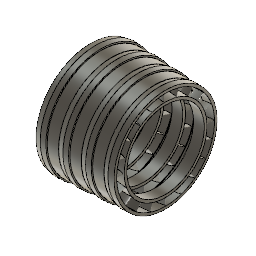
Untitled v3 (Autodesk Fusion 360 design; units mm, degrees)
Autodesk Fusion 360 part; units mm, degrees
note: some values were not read from the file. Chosen so that the rebuilt part matches the saved one: which bodies a step acts on.
sketch "Sketch1" plane through (0, 0, 0) normal (0, 1, 0) x (1, 0, 0)
  line L0 (0, -72.01) -> (20, -72.01)
  line L1 (40, -72.01) -> (60, -72.01)
  line L2 (80, -72.01) -> (100, -72.01)
  line L3 (120, -72.01) -> (140, -72.01)
  line L4 (120, -77.01) -> (140, -77.01)
  line L5 (80, -77.01) -> (100, -77.01)
  line L6 (40, -77.01) -> (60, -77.01)
  line L7 (0, -77.01) -> (20, -77.01)
  line L8 (0, -72.01) -> (234.5809, -72.01) construction
  line L9 (0, -72.01) -> (0, -77.01)
  line L10 (20, -72.01) -> (20, -77.01)
  line L11 (40, -72.01) -> (40, -77.01)
  line L12 (60, -72.01) -> (60, -77.01)
  line L13 (80, -72.01) -> (80, -77.01)
  line L14 (100, -72.01) -> (100, -77.01)
  line L15 (120, -72.01) -> (120, -77.01)
  line L16 (140, -72.01) -> (140, -77.01)
  line L17 (0, -98.8982) -> (0, -101.4021)
  line L18 (40, -96.6619) -> (40, -98.1642)
  line L19 (80, -94.4255) -> (80, -95.9279)
  line L20 (120, -92.1892) -> (120, -93.6915)
  line L21 (140, -91.071) -> (140, -121.2503)
  line L22 (140, -96.0788) -> (129.3625, -96.6736)
  line L23 (140.0185, -91.07) -> (120, -92.1892)
  line L24 (100, -98.3152) -> (90, -98.8743)
  line L25 (100, -93.3074) -> (80, -94.4255)
  line L26 (60, -100.5515) -> (50, -101.1106)
  line L27 (20, -102.7879) -> (10, -103.347)
  line L28 (60, -95.5437) -> (39.9, -96.6675)
  line L29 (20, -97.7801) -> (0, -98.8982)
  line L30 (0, 0) -> (0, -77.01) construction
  line L31 (0, -98.8982) -> (0, -101.4021) construction
  line L32 (10, -103.347) -> (0, -101.4021)
  line L33 (129.3625, -96.6736) -> (129.374, -96.6736)
  line L34 (129.374, -96.6736) -> (120, -94.6931)
  line L35 (90, -98.8743) -> (80, -96.9295)
  line L36 (50, -101.1106) -> (40, -99.1658)
  line L37 (20, -100.284) -> (40, -99.1658)
  line L38 (20, -99.2824) -> (40, -98.1642)
  line L39 (60, -98.0476) -> (80, -96.9295)
  line L40 (100, -95.8113) -> (120, -94.6931)
  line L41 (60, -97.0461) -> (80, -95.9279)
  line L42 (100, -94.8097) -> (119.9442, -93.6947)
  line L43 (100, -93.3074) -> (100, -94.8097)
  line L44 (100, -95.8113) -> (100, -115.1614)
  line L45 (119.9442, -93.6947) -> (120, -93.6915)
  line L46 (60, -95.5437) -> (60, -97.0461)
  line L47 (60, -98.0476) -> (60, -117.9989)
  line L48 (20, -97.7801) -> (20, -99.2824)
  line L49 (20, -100.284) -> (20, -102.7879)
  point P0 (160, -72.01)
  dimension "d2" = 20
  dimension "d3" = 20
  dimension "d4" = 20
  dimension "d5" = 20
  dimension "d6" = 20
  dimension "d7" = 20
  dimension "d8" = 20
  dimension "d9" = 5
  dimension "d10" = 5
  dimension "d11" = 5
  dimension "d12" = 5
  dimension "d13" = 234.5809
  dimension "d14" = 72.01
  dimension "d15" = 19.06
  dimension "d16" = 20
  dimension "d17" = 3.2
  constraint coincident L30.start origin
  constraint vertical L30
  constraint coincident L0.start L30
  constraint perpendicular L0 L30
  constraint perpendicular L8 L30
  constraint coincident L17.start L30
  constraint coincident L8 P0
  constraint coincident L29.start L23
  constraint coincident L27.start L22
  constraint parallel L10 L48
  constraint coincident L28.end L23
  constraint perpendicular L6 L18
  constraint perpendicular L6 L46
  constraint perpendicular L5 L19
  constraint perpendicular L5 L43
  constraint perpendicular L4 L20
  constraint perpendicular L4 L21
  constraint coincident L21 L22.start
  constraint coincident L24.start L43
  constraint collinear L22 L24
  constraint collinear L23 L25
  constraint coincident L26.start L46
  constraint collinear L24 L26
  constraint collinear L25 L28
  constraint collinear L26 L27
  constraint collinear L28 L29
  constraint collinear L30 L31
  constraint coincident L28 L18.start
  constraint coincident L23 L21.start
  constraint perpendicular L20 L33
  constraint coincident L35.end L39.end
  constraint coincident L36.end L37.end
  constraint parallel L35 L36
  constraint coincident L37.start L48
  constraint coincident L39.start L46
  constraint collinear L37 L39
  constraint collinear L38 L41
  constraint coincident L40.start L43
  constraint collinear L39 L40
  constraint collinear L41 L42
  constraint collinear L43 L44
  constraint parallel L42 L45
  constraint collinear L46 L47
  constraint collinear L48 L49
  measures "d2" distance of L0.start L0.end
  measures "d3" distance of L1.start L1.end
  measures "d4" distance of L2.start L2.end
  measures "d5" distance of L3.start L3.end
  measures "d6" distance of L0.end L1.start
  measures "d7" distance of L1.end L2.start
  measures "d8" distance of L2.end L3.start
  measures "d13" distance of L0.start L8.end
  measures "d14" distance of L30.start L8
  measures "d15" distance of L3.end L23.start
  measures "d16" distance of L3.end P0
  measures "d17" angle of L0 L23
revolve "Revolve1" add sketch "Sketch1" angle 360 about axis through (1.75, 0, 0) along (1, 0, 0) makes body 1 at (86.6667, 3.8386, 76.9143) makes body 2 at (46.6667, 3.8386, 76.9143) makes body 3 at (126.6667, 3.8386, 76.9143) makes body 4 at (6.6667, 3.8386, 76.9143) makes body 5 at (26.6667, 4.9802, 99.7871)
sketch "Sketch2" plane through (0, 0, 0) normal (0, 0, 1) x (1, 0, 0)
  ellipse E0 centre (10, 0) end of major axis (18.8633, -1.5628) minor radius 1
  line L0 (1.1367, 1.5628) -> (18.8633, -1.5628) construction
  line L1 (9.8264, -0.9848) -> (10.1736, 0.9848) construction
  line L2 (0, 0) -> (202.6792, 0) construction
  ellipse E1 centre (50, 0) end of major axis (58.8633, -1.5628) minor radius 1
  line L3 (41.1367, 1.5628) -> (58.8633, -1.5628) construction
  line L4 (49.8264, -0.9848) -> (50.1736, 0.9848) construction
  ellipse E2 centre (90, 0) end of major axis (98.8633, -1.5628) minor radius 1
  line L5 (81.1367, 1.5628) -> (98.8633, -1.5628) construction
  line L6 (89.8264, -0.9848) -> (90.1736, 0.9848) construction
  ellipse E3 centre (129.3716, 0) end of major axis (138.2348, -1.5628) minor radius 1
  line L7 (120.5083, 1.5628) -> (138.2348, -1.5628) construction
  line L8 (129.1979, -0.9848) -> (129.5452, 0.9848) construction
  point P0 (10, 0)
  point P1 (50, 0)
  point P2 (90, 0)
  point P3 (129.3716, 0)
  dimension "d27" = 18
  dimension "d28" = 2
  dimension "d29" = 10
  dimension "d30" = 18
  dimension "d31" = 2
  dimension "d32" = 10
  dimension "d33" = 18
  dimension "d34" = 2
  dimension "d35" = 10
  dimension "d36" = 18
  dimension "d37" = 2
  dimension "d38" = 10
  constraint coincident E0 L0.start
  constraint coincident E0 L0.end
  constraint coincident E0 L1.start
  constraint coincident E0 L1.end
  constraint coincident P0 E0.centre
  constraint coincident L2.start origin
  constraint horizontal L2
  constraint coincident E1 L3.start
  constraint coincident E1 L3.end
  constraint coincident E1 L4.start
  constraint coincident E1 L4.end
  constraint coincident P1 E1.centre
  constraint coincident E2 L5.start
  constraint coincident E2 L5.end
  constraint coincident E2 L6.start
  constraint coincident E2 L6.end
  constraint coincident P2 E2.centre
  constraint coincident E3 L7.start
  constraint coincident E3 L7.end
  constraint coincident E3 L8.start
  constraint coincident E3 L8.end
  constraint coincident P3 E3.centre
  measures "d27" distance of E0
  measures "d29" angle of L0 L2
  measures "d30" distance of E1
  measures "d32" angle of L2 L3
  measures "d33" distance of E2
  measures "d35" angle of L2 L5
  measures "d36" distance of E3
  measures "d38" angle of L2 L7
extrude "Extrude1" add sketch "Sketch2" along normal blind 100 separate body contours E0 makes body 6
extrude "Extrude2" add sketch "Sketch2" along normal blind 98 separate body contours E1 makes body 7
extrude "Extrude3" add sketch "Sketch2" along normal blind 95.8 separate body contours E2 makes body 8
extrude "Extrude4" add sketch "Sketch2" along normal blind 91 separate body contours E3 makes body 9
pattern_circular "C-Pattern1" count 20 over 360 about axis through (0, 0, 0) along (1, 0, 0) of bodies 6 7 8 9 makes body 10 at (9.3321, -24.0343, 77.6221) makes body 11 at (6.5283, -37.941, 54.8388) makes body 12 at (6.5283, -26.0629, 20.8375) makes body 13 at (9.3321, -17.4835, 6.8674) makes body 14 at (8.7492, -85.4167, -0.7873) makes body 15 at (9.3321, -77.6221, -24.0343) makes body 16 at (6.5283, -54.8388, -37.941) makes body 17 at (6.5283, -40.4304, -53.0302) makes body 18 at (9.3321, -26.181, -76.9246) makes body 19 at (8.7492, 0.7873, -85.4167) makes body 20 at (9.3321, 24.0343, -77.6221) makes body 21 at (6.5283, 37.941, -54.8388) makes body 22 at (6.5283, 26.0629, -20.8375) makes body 23 at (9.3321, 17.4835, -6.8674) makes body 24 at (8.7492, 85.4167, 0.7873) makes body 25 at (9.3321, 77.6221, 24.0343) makes body 26 at (6.5283, 54.8388, 37.941) makes body 27 at (6.5283, 40.4304, 53.0302) makes body 28 at (9.3321, 6.8674, 17.4835) makes body 29 at (49.4552, -23.5516, 76.0703) makes body 30 at (49.3747, -9.8932, 15.5249) makes body 31 at (49.3747, -63.7587, 47.7098) makes body 32 at (49.4552, -75.3854, 25.6594) makes body 33 at (51.017, -91.3646, 0.8315) makes body 34 at (49.4552, -76.0703, -23.5516) makes body 35 at (49.3747, -65.0772, -45.895) makes body 36 at (49.3747, -47.7098, -63.7587) makes body 37 at (49.4552, -25.6594, -75.3854) makes body 38 at (51.017, -0.8315, -91.3646) makes body 39 at (49.4552, 23.5516, -76.0703) makes body 40 at (49.3747, 9.8932, -15.5249) makes body 41 at (49.3747, 63.7587, -47.7098) makes body 42 at (49.4552, 75.3854, -25.6594) makes body 43 at (51.017, 91.3646, -0.8315) makes body 44 at (49.4552, 17.8181, 4.6243) makes body 45 at (49.3747, 15.5249, 9.8932) makes body 46 at (49.3747, 11.7079, 14.2065) makes body 47 at (49.4552, 25.6594, 75.3854) makes body 48 at (89.7455, -9.9815, 27.5792) makes body 49 at (91.6749, -4.5618, 4.0866) makes body 50 at (91.6749, -5.6014, 2.4769) makes body 51 at (89.7455, -63.532, 19.6224) makes body 52 at (89.2673, -41.9125, 1.1393) makes body 53 at (89.7455, -27.5792, -9.9815) makes body 54 at (91.6749, -71.9025, -53.8329) makes body 55 at (91.6749, -2.4769, -5.6014) makes body 56 at (89.7455, -8.1355, -28.179) makes body 57 at (89.2673, -1.1393, -41.9125) makes body 58 at (89.7455, 9.9815, -27.5792) makes body 59 at (91.6749, 53.8329, -71.9025) makes body 60 at (91.6749, 73.4172, -51.748) makes body 61 at (89.7455, 63.532, -19.6224) makes body 62 at (89.2673, 41.9125, -1.1393) makes body 63 at (89.7455, 62.9322, 21.4684) makes body 64 at (91.6749, 71.9025, 53.8329) makes body 65 at (91.6749, 51.748, 73.4172) makes body 66 at (89.7455, 8.1355, 28.179) makes body 67 at (129.0882, -10.7049, 36.3897) makes body 68 at (129.2032, -30.3567, 43.5592) makes body 69 at (129.2032, -42.3315, 32.0465) makes body 70 at (129.0882, -50.1564, 17.4156) makes body 71 at (129.0958, -53.0833, 1.0627) makes body 72 at (129.0882, -36.3897, -10.7049) makes body 73 at (129.2032, -43.5592, -30.3567) makes body 74 at (129.2032, -32.0465, -42.3315) makes body 75 at (129.0882, -17.4156, -50.1564) makes body 76 at (129.0958, -1.0627, -53.0833) makes body 77 at (129.0882, 10.7049, -36.3897) makes body 78 at (129.2032, 21.442, -31.2891) makes body 79 at (129.2032, 42.3315, -32.0465) makes body 80 at (129.0882, 50.1564, -17.4156) makes body 81 at (129.0958, 53.0833, -1.0627) makes body 82 at (129.0882, 50.8141, 15.3917) makes body 83 at (129.2032, 43.5592, 30.3567) makes body 84 at (129.2032, 32.0465, 42.3315) makes body 85 at (129.0882, 17.4156, 50.1564)
sketch "Sketch3" plane through (0, 0, 0) normal (-1, 0, 0) x (0, -1, 0)
  circle A0 centre (0, 0) radius 77.01
  circle A1 centre (0, 0) radius 72.01
  circle A2 centre (0, 0) radius 72.01
  dimension "d49" = 144.02
  constraint coincident A0.centre A1.centre
  measures "d49" diameter of A2
extrude "Extrude5" cut sketch "Sketch3" along normal mid plane 400 contours A1 A2 bodies 6 7 8 9 10 11 12 13 14 15 16 17 18 19 20 21 22 23 24 25 26 27 28 29 30 31 32 33 34 35 36 37 38 39 40 41 42 43 44 45 46 47 48 49 50 51 52 53 54 55 56 57 58 59 60 61 62 63 64 65 66 67 68 69 70 71 72 73 74 75 76 77 78 79 80 81 82 83 84 85
combine "Combine1" operation add target body 5 tool bodies 3 67 11 17 2 1 4 21 29 57 72 75 82 80 44 30 62 60 24 16 56 35 38 70 13 51 84 63 34 79 19 7 48 10 45 59 26 74 22 20 54 27 40 78 25 9 53 28 64 73 81 37 43 61 15 32 6 76 49 83 23 66 52 71 77 14 58 47 46 65 41 68 18 50 12 55 8 31 39 69 85 36 42 33 makes body 86 at (127.8088, -12.133, 76.0482)
